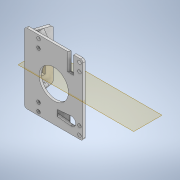
# Autodesk Inventor part: base_v3_door_v3-4
Saved by Autodesk Inventor 2021 (Build 250183000, 183)
## iProperties
Created: 2023-04-16
Part Number: base_v3_door_v3-4
Material: Generic
Document SubType Name: Modeling
Designer: malo
Density: 1 g/cm^3
Appearance: Default
Author: malo
Autodesk Inventor part; units mm, degrees
ref_plane "YZ Plane" through (0, 0, 0) normal (1, 0, 0) x (0, 1, 0)
ref_plane "XZ Plane" through (0, 0, 0) normal (0, 1, 0) x (-1, 0, 0)
ref_plane "XY Plane" through (0, 0, 0) normal (0, 0, 1) x (1, 0, 0)
sketch "Sketch1" plane through (0, 0, 0) normal (0, 0, 1) x (1, 0, 0)
  line L0 (0, 0) -> (50, 0)
  line L1 (50, 0) -> (50, 60)
  line L2 (50, 60) -> (0, 60)
  line L3 (0, 60) -> (0, 0)
  dimension "d0" = 50
  dimension "d1" = 60
  constraints: 8 end point, 2 parallel, 1 horizontal, 1 perpendicular
  measures "d0" distance of L2.end L1.end
  measures "d1" distance of L1.end L0.end
extrude "Extrusion1" add sketch "Sketch1" along normal blind 2
sketch "Sketch3" plane through (0, 0, 0) normal (-1, 0, 0) x (0, 0, 1)
  line L0 (0, 60) -> (0, 0) projected
  line L1 (0, 0) -> (0, 60) projected
  line L2 (0, 56) -> (-20, 51)
  line L3 (-20, 51) -> (-20, 9)
  line L4 (-20, 9) -> (0, 4)
  line L5 (0, 18.5) -> (-13, 18.5)
  line L6 (-13, 18.5) -> (-13, 41.5)
  line L7 (-13, 41.5) -> (0, 41.5)
  line L8 (0, 41.5) -> (0, 18.5)
  line L9 (0, 60) -> (2, 60) projected
  circle A0 centre (-6.5, 43.25) radius 1
  circle A1 centre (-6.5, 16.75) radius 1
  point P0 (0, 41.5)
  point P1 (-13, 30)
  dimension "d15" = 20
  dimension "d16" = 13
  dimension "d17" = 23
  dimension "d18" = 18.5
  dimension "d19" = 2
  dimension "d20" = 2
  dimension "d21" = 6.5
  dimension "d22" = 6.5
  dimension "d25" = 5
  dimension "d45" = 4
  dimension "d46" = 4
  dimension "d72" = 13.25
  dimension "d73" = 13.25
  dimension "d100" = 5
  constraints: 14 end point, 3 parallel, 3 point on line, 2 centre point, 1 horizontal, 1 midpoint, 1 perpendicular
  measures "d15" distance between parallel lines of L3 L0
  measures "d16" distance of L5.start L5.end
  measures "d17" distance of L5.end L6.end
  measures "d18" distance between parallel lines of L9 L7
  measures "d19" diameter of A0
  measures "d20" diameter of A1
  measures "d21" distance from line of A0.centre L0
  measures "d22" distance from line of L0 A1.centre
  measures "d25" vertical distance of L2.start L2.end
  measures "d45" distance of L0.end L4.end
  measures "d46" distance from line of L9 L2.start
  measures "d72" vertical distance of point (-13, 30) A0.centre
  measures "d73" vertical distance of point (-13, 30) A1.centre
  measures "d100" vertical distance of L3.end L4.end
extrude "Extrusion3" add sketch "Sketch3" against normal blind 2.5 contours L0 L7 L6 L5 L4 L3 L2
sketch "Sketch8" plane through (0, 0, 0) normal (0, 0, -1) x (-1, 0, 0)
  line L0 (-2.5, 56) -> (0, 56) projected
  line L1 (0, 56) -> (0, 41.5) projected
  line L2 (0, 41.5) -> (-2.5, 41.5) projected
  line L3 (0, 41.5) -> (0, 18.5) projected
  line L4 (0, 18.5) -> (0, 4) projected
  line L5 (0, 4) -> (-2.5, 4) projected
  line L6 (-2.5, 18.5) -> (0, 18.5) projected
  line L7 (-2.5, 41.5) -> (-2.5, 53)
  line L8 (-2.5, 53) -> (-6.5, 47)
  circle A0 centre (-5.5, 47) radius 1
  line L9 (0, 0) -> (-50, 0) projected
  line L10 (-50, 60) -> (0, 60) projected
  line L11 (0, 60) -> (0, 56) projected
  line L12 (0, 4) -> (0, 0) projected
  line L13 (-50, 0) -> (-50, 60) projected
  line L14 (-2.5, 41.5) -> (-2.5, 56) projected
  line L15 (-2.5, 4) -> (-2.5, 18.5) projected
  line L16 (-6.5, 47) -> (-2.5, 47)
  line L17 (-2.5, 41.5) -> (-2.5, 56) projected
  point P0 (-5.8846, 47.9231)
  point P1 (-4.5, 47)
  point P2 (-2.5, 47)
  dimension "d75" = 6
  dimension "d77" = 2
  dimension "d78" = 1
  dimension "d98" = 5.5
  dimension "d99" = 4
  constraints: 6 end point, 2 point on line, 1 centre point, 1 perpendicular, 1 vertical
  measures "d75" vertical distance of L7.end L8.end
  measures "d77" diameter of A0
  measures "d78" distance of L8.end A0.centre
  measures "d98" distance between parallel lines of L2 L16
  measures "d99" distance of L8.end L16.end
extrude "Extrusion8" add sketch "Sketch8" along normal blind 12 contours L7 L16 A0 L8 | A0 L16 L8 | L8 A0 | A0 L16
ref_plane "Work Plane4" through (0, 30, 0) normal (0, 1, 0) x (1, 0, 0)
mirror "Mirror3" about plane through (0, 30, 0) normal (0, 1, 0) of "Extrusion8"
fillet "Fillet6" radius 2 2 edges at (1.25, 51, -20) (1.25, 9, -20)
sketch "Sketch15" plane through (0, 0, 2) normal (0, 0, 1) x (1, 0, 0)
  circle A0 centre (40, 10) radius 3.75
  line L0 (0, 0) -> (50, 0) projected
  line L1 (0, 60) -> (0, 0) projected
  circle A1 centre (24.5, 10) radius 2.25
  line L2 (40, 10) -> (69.4613, 10) construction
  line L3 (24.5, 7.75) -> (24.5, 12.25) construction
  line L4 (24.5, 7.75) -> (39.6345, 6.2679)
  line L5 (24.5, 12.25) -> (39.6345, 13.7321)
  dimension "d135" = 7.5
  dimension "d136" = 10
  dimension "d137" = 40
  dimension "d138" = 4.5
  dimension "d145" = 15.5
  constraints: 8 end point, 4 point on circle, 2 centre point, 2 tangent, 1 horizontal, 1 midpoint, 1 point on line, 1 vertical
  measures "d135" diameter of A0
  measures "d136" distance from line of L0 L2.start
  measures "d137" distance from line of L1 L2.start
  measures "d138" diameter of A1
  measures "d145" distance of A1.centre L2.start
extrude "Extrusion15" cut sketch "Sketch15" against normal blind 2
sketch "Sketch20" plane through (0, 0, 0) normal (0, 0, -1) x (-1, 0, 0)
  line L0 (-39.6345, 6.2679) -> (-24.5, 7.75) projected
  arc A0 (-24.5, 7.75) -> (-24.5, 12.25) centre (-24.5, 10) ccw projected
  line L1 (-24.5, 12.25) -> (-39.6345, 13.7321) projected
  arc A1 (-39.6345, 13.7321) -> (-39.6345, 6.2679) centre (-40, 10) ccw projected
  line L2 (0, 0) -> (-50, 0) projected
  line L3 (-50, 0) -> (-50, 60) projected
  line L4 (-50, 60) -> (0, 60) projected
  line L5 (0, 60) -> (0, 56) projected
  line L6 (0, 56) -> (0, 41.5) projected
  line L7 (0, 41.5) -> (0, 18.5) projected
  line L8 (0, 18.5) -> (0, 4) projected
  line L9 (0, 4) -> (0, 0) projected
  line L10 (-2.5, 56) -> (0, 56) projected
  line L11 (-2.5, 53) -> (-2.5, 56) projected
  line L12 (-5.8846, 47.9231) -> (-2.5, 53) projected
  arc A2 (-5.8846, 47.9231) -> (-4.5, 47) centre (-5.5, 47) ccw projected
  line L13 (-2.5, 47) -> (-4.5, 47) projected
  line L14 (-2.5, 41.5) -> (-2.5, 47) projected
  line L15 (0, 41.5) -> (-2.5, 41.5) projected
  line L16 (-2.5, 18.5) -> (0, 18.5) projected
  line L17 (-2.5, 13) -> (-2.5, 18.5) projected
  line L18 (-4.5, 13) -> (-2.5, 13) projected
  arc A3 (-4.5, 13) -> (-5.8846, 12.0769) centre (-5.5, 13) ccw projected
  line L19 (-2.5, 7) -> (-5.8846, 12.0769) projected
  line L20 (-2.5, 4) -> (-2.5, 7) projected
  line L21 (0, 4) -> (-2.5, 4) projected
  line L22 (-24.5, 12.25) -> (-39.6345, 13.7321) projected
  line L23 (-36, 14.381) -> (-36, 5.619)
  line L24 (-24.5, 7.75) -> (-39.6345, 6.2679) projected
  arc A4 (-24.5, 6.75) -> (-24.5, 13.25) centre (-24.5, 10) ccw
  line L25 (-24.4025, 13.2452) -> (-39.537, 14.7274)
  line L26 (-39.537, 5.2726) -> (-24.4025, 6.7548)
  point P0 (-36, 13.3762)
  point P1 (-36, 6.6238)
  point P2 (-24.4467, 6.7504)
  point P3 (-24.4467, 13.2496)
  dimension "d165" = 4
  dimension "d171" = 1
  dimension "d172" = 1
  dimension "d173" = 1
  constraints: 6 end point, 2 parallel, 2 point on circle, 2 point on line, 1 centre point, 1 vertical
  measures "d165" distance from line of A1.centre L23
  measures "d171" radial gap between concentric circles of A0 A4
  measures "d172" distance between parallel lines of L1 L25
  measures "d173" distance between parallel lines of L0 L26
extrude "Extrusion20" add sketch "Sketch20" along normal blind 1 contours L23 L1 A0 L0 | L0 A0 L1 L23 L25 A4 L26
sketch "Sketch21" plane through (0, 0, 2) normal (0, 0, 1) x (1, 0, 0)
  line L0 (24.5, 7.75) -> (39.6345, 6.2679) projected
  arc A0 (39.6345, 6.2679) -> (39.6345, 13.7321) centre (40, 10) ccw projected
  line L1 (39.6345, 13.7321) -> (24.5, 12.25) projected
  arc A1 (24.5, 12.25) -> (24.5, 7.75) centre (24.5, 10) ccw projected
  line L2 (50, 0) -> (0, 0) projected
  line L3 (0, 0) -> (0, 60) projected
  line L4 (0, 60) -> (50, 60) projected
  line L5 (50, 60) -> (50, 0) projected
  line L6 (39.6345, 6.2679) -> (24.5, 7.75) projected
  line L7 (28, 7.4072) -> (28, 12.5928)
  line L8 (24.5, 12.25) -> (39.6345, 13.7321) projected
  dimension "d168" = 3.5
  constraints: 2 end point, 2 point on line, 1 vertical
  measures "d168" distance from line of A1.centre L7
extrude "Extrusion21" add sketch "Sketch21" against normal blind 0.5 contours A1 L1 L7 L0
chamfer "Chamfer5" distance 1 angle 45 3 edges at (30.2233, 6.1847, 0) (21.25, 10, 0) (30.2233, 13.8153, 0)
sketch "Sketch14" plane through (0, 0, 0) normal (0, 0, -1) x (-1, 0, 0)
  circle A0 centre (-47, 3) radius 1.5
  line L0 (-50, 0) -> (-50, 60) projected
  line L1 (0, 0) -> (-50, 0) projected
  circle A1 centre (-47, 10) radius 1.5
  dimension "d127" = 3
  dimension "d128" = 3
  dimension "d129" = 3
  dimension "d130" = 3
  dimension "d131" = 3
  dimension "d132" = 10
  constraints: 2 centre point
  measures "d127" diameter of A0
  measures "d128" distance from line of L0 A0.centre
  measures "d129" distance from line of L1 A0.centre
  measures "d130" diameter of A1
  measures "d131" distance from line of L0 A1.centre
  measures "d132" distance from line of L1 A1.centre
extrude "Extrusion14" cut sketch "Sketch14" against normal blind 14
mirror "Mirror4" about plane through (0, 30, 0) normal (0, 1, 0) of "Extrusion14"
sketch "Sketch17" plane through (0, 0, 0) normal (0, 0, -1) x (-1, 0, 0)
  circle A0 centre (-25, 30) radius 12.5
  line L0 (0, 0) -> (-50, 0) projected
  line L1 (-50, 0) -> (-50, 60) projected
  dimension "d146" = 30
  dimension "d147" = 25
  dimension "d148" = 25
  constraints: 1 centre point
  measures "d146" distance from line of L0 A0.centre
  measures "d147" distance from line of L1 A0.centre
  measures "d148" diameter of A0
extrude "Extrusion17" cut sketch "Sketch17" against normal blind 2
sketch "Sketch18" plane through (0, 0, 0) normal (0, 0, -1) x (-1, 0, 0)
  circle A0 centre (-18, 3) radius 1.25
  line L0 (0, 0) -> (-50, 0) projected
  line L1 (0, 4) -> (0, 0) projected
  dimension "d152" = 2.5
  dimension "d153" = 3
  dimension "d154" = 18
  constraints: 1 centre point
  measures "d152" diameter of A0
  measures "d153" distance from line of L0 A0.centre
  measures "d154" distance from line of L1 A0.centre
extrude "Extrusion18" add sketch "Sketch18" along normal blind 2.5
sketch "Sketch19" plane through (0, 0, 0) normal (0, 0, -1) x (-1, 0, 0)
  line L0 (0, 4) -> (-2.5, 4) projected
  line L1 (-2.5, 13) -> (-2.5, 7) projected
  line L2 (0, 4) -> (-2.5, 4)
  line L3 (-2.5, 4) -> (-2.5, 7)
  line L4 (-3.1667, 8) -> (0, 8)
  line L5 (0, 8) -> (0, 4)
  line L6 (-2.5, 7) -> (-5.8846, 12.0769) projected
  point P0 (0, 0)
  dimension "d161" = 4
  constraints: 8 end point, 2 parallel, 2 point on line, 1 horizontal, 1 perpendicular
  measures "d161" distance of L4.end L0.start
extrude "Extrusion19" cut sketch "Sketch19" along normal blind 2
sketch "Sketch22" plane through (0, 60, 0) normal (0, 1, 0) x (1, 0, 0)
  line L0 (50, 0) -> (0, 0) projected
  line L1 (0, 0) -> (0, -2) projected
  line L2 (50, -2) -> (0, -2) projected
  line L3 (50, 0) -> (50, -2) projected
  line L4 (50, -2) -> (0, -2) projected
  line L5 (36.8, -2) -> (37.9547, 0)
  line L6 (0, 0) -> (50, 0) projected
  line L7 (36.8, -2) -> (42, -2)
  line L8 (42, -2) -> (42, 0)
  line L9 (37.9547, 0) -> (42, 0)
  line L10 (50, 0) -> (0, 0) projected
  point P0 (37.9547, 0)
  point P1 (36.8, -2)
  dimension "d183" = 60
  dimension "d184" = 5.2
  dimension "d185" = 8
  constraints: 8 end point, 4 point on line, 1 collinear, 1 perpendicular
  measures "d183" angle of L2 L5
  measures "d184" distance of L5.start L7.end
  measures "d185" distance between parallel lines of L3 L8
extrude "Extrusion22" cut sketch "Sketch22" against normal blind 15 contours L8 L2 L5 L0
fillet "Fillet9" radius 1 1 edges at (1.25, 4.5, -2)
fillet "Fillet7" radius 2 4 edges at (50, 60, 1) (0, 60, 1) (50, 0, 1) (0, 0, 1)
fillet "Fillet8" radius 1 1 edges at (19.25, 3, -2.5)
move faces "Move1" translate (0, 0, -0.5) faces at (32.1667, 9.25, 0)
pattern_linear "Rectangular Pattern1" count 2 spacing 35 along (-1, 0, 0) of "Extrusion14", "Mirror4"
equation "\"d20\" = d19"
equation "\"d21\" = 0.5 * d16"
equation "\"d22\" = d21"
body "Solid1"
